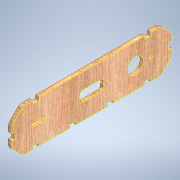
# Autodesk Inventor part: side
Saved by Autodesk Inventor 2020 (Build 240168000, 168)
## iProperties
Created: 2020-02-17
Part Number: side
Material: Wood (Birch)
Document SubType Name: Modeling
Designer: erwin
Density: 0.55 g/cm^3
Appearance: Birch - Natural Polished
Author: erwin
Autodesk Inventor part; units mm, degrees
ref_plane "YZ Plane" through (0, 0, 0) normal (1, 0, 0) x (0, 1, 0)
ref_plane "XZ Plane" through (0, 0, 0) normal (0, 1, 0) x (-1, 0, 0)
ref_plane "XY Plane" through (0, 0, 0) normal (0, 0, 1) x (1, 0, 0)
sketch "Sketch1" plane through (0, 0, 0) normal (1, 0, 0) x (0, 1, 0)
  line L0 (37.5736, 300) -> (-37.5736, 300)
  line L1 (-37.5736, 300) -> (-80, 257.5736)
  line L2 (-80, 257.5736) -> (-80, -257.5736)
  line L3 (-80, -257.5736) -> (-37.5736, -300)
  line L4 (-37.5736, -300) -> (37.5736, -300)
  line L5 (80, 257.5736) -> (80, -257.5736)
  line L6 (13.6652, 0) -> (-15.1656, 0) construction
  line L7 (0, 10.5835) -> (0, -18.7754) construction
  circle A0 centre (0, -220) radius 6
  line L8 (-0.0152, 220) -> (-0.0152, 180) construction
  line L9 (-6.0152, 220) -> (-6.0152, 180)
  line L10 (5.9848, 180) -> (5.9848, 220)
  arc A1 (5.9848, 220) -> (-6.0152, 220) centre (-0.0152, 220) ccw
  arc A2 (-6.0152, 180) -> (5.9848, 180) centre (-0.0152, 180) ccw
  line L11 (37.5736, 300) -> (80, 257.5736)
  line L12 (80, -257.5736) -> (37.5736, -300)
  circle A3 centre (-0.0152, -164) radius 30
  point P0 (0, 0)
  point P1 (80, 300)
  point P2 (80, -300)
  point P3 (-0.0152, 200)
  dimension "d0" = 160
  dimension "d1" = 45
  dimension "d2" = 12
  dimension "d3" = 40
  dimension "d4" = 12
  dimension "d5" = 400
  dimension "d6" = 80
  dimension "d7" = 80
  dimension "d8" = 80
  dimension "d9" = 80
  dimension "d10" = 60
  dimension "d15" = 60
  dimension "d16" = 60
  dimension "d17" = 45
  dimension "d18" = 56
  dimension "d19" = 60
  constraints: 28 end point, 4 centre point, 4 point on circle, 4 point on line, 4 tangent, 3 horizontal, 2 equal length, 2 parallel, 2 perpendicular, 2 vertical, 1 midpoint, 2 other
  measures "d0" distance between parallel lines of L5 L2
  measures "d1" angle of L4 L3
  measures "d2" diameter of A0
  measures "d3" distance of L8.start L8.end
  measures "d4" diameter of A2
  measures "d5" distance of A0.centre L8.end
  measures "d6" distance from line of L5 A0.centre
  measures "d7" distance from line of A0.centre L4
  measures "d8" distance from line of L2 A0.centre
  measures "d9" distance from line of L0 L8.start
  measures "d10" distance of L0.end L1.end
  measures "d15" distance of L0.start L5.start
  measures "d16" distance of L5.end L4.end
  measures "d17" angle of L5 L12
  measures "d18" distance of A0.centre A3.centre
  measures "d19" diameter of A3
extrude "Extrusion1" add sketch "Sketch1" along normal blind 12
fillet "Fillet1" radius 24 2 edges at (6, 80, 257.5736) (6, 37.5736, 300)
mirror "Mirror1" about plane through (0, 0, 0) normal (0, 1, 0) of "Fillet1"
mirror "Mirror2" about plane through (0, 0, 0) normal (0, 0, 1) of "Fillet1", "Mirror1"
sketch "Sketch6" plane through (0, 80, 247.6325) normal (0, 1, 0) x (1, 0, 0)
  line L0 (0, 67.6325) -> (0, 27.6325) projected
  line L1 (0, 50.07) -> (12, 50.07)
  line L2 (12, 50.07) -> (12, 26.07)
  line L3 (12, 26.07) -> (0, 26.07)
  line L4 (0, 26.07) -> (0, 50.07)
  point P0 (0, 247.6325)
  dimension "d23" = 12
  dimension "d24" = 24
  constraints: 8 end point, 2 parallel, 1 horizontal, 1 perpendicular, 1 point on line
  measures "d23" distance of L2.end L3.end
  measures "d24" distance of L1.end L2.end
extrude "Extrusion2" cut sketch "Sketch6" against normal blind 12
sketch "Sketch7" plane through (0, 27.6325, 300) normal (0, 0, 1) x (1, 0, 0)
  line L0 (-12, -15.6325) -> (12, -15.6325)
  line L1 (12, -15.6325) -> (12, -39.6325)
  line L2 (12, -39.6325) -> (-12, -39.6325)
  line L3 (-12, -39.6325) -> (-12, -15.6325)
  line L4 (-12, -15.6325) -> (12, -39.6325) construction
  line L5 (12, -15.6325) -> (-12, -39.6325) construction
  point P0 (0, -27.6325)
  dimension "d27" = 24
  dimension "d28" = 24
  constraints: 12 end point, 2 midpoint, 2 parallel, 1 horizontal, 1 perpendicular
  measures "d27" distance of L1.end L2.end
  measures "d28" distance of L0.end L1.end
extrude "Extrusion3" cut sketch "Sketch7" against normal blind 12
mirror "Mirror3" about plane through (0, 0, 0) normal (0, 1, 0) of "Extrusion2"
mirror "Mirror4" about plane through (0, 0, 0) normal (0, 0, 1) of "Extrusion2", "Mirror3", "Extrusion3"
sketch "Sketch8" plane through (0, -80, 197.5625) normal (0, -1, 0) x (1, 0, 0)
  line L0 (12, 0) -> (12, -395.125) projected
  line L1 (0, 0) -> (0, -395.125) projected
  line L2 (12, -115.7083) -> (0, -115.7083)
  line L3 (0, -115.7083) -> (0, -139.7083)
  line L4 (0, -139.7083) -> (12, -139.7083)
  line L5 (12, -139.7083) -> (12, -115.7083)
  line L6 (12, 0) -> (0, 0) projected
  line L7 (0, -395.125) -> (12, -395.125) projected
  point P0 (0, -197.5625)
  dimension "d31" = 24
  dimension "d32" = 115.7083
  dimension "d33" = 255.4167
  constraints: 8 end point, 2 parallel, 2 point on line, 1 horizontal, 1 perpendicular
  measures "d31" distance of L3.end L2.end
  measures "d32" distance between parallel lines of L6 L2
  measures "d33" distance between parallel lines of L7 L4
extrude "Extrusion4" cut sketch "Sketch8" against normal blind 12 contours L0 L4 L1 L2
mirror "Mirror5" about plane through (0, 0, 0) normal (0, 0, 1) of "Extrusion4"
sketch "Sketch9" plane through (12, 0, 0) normal (1, 0, 0) x (0, 0, -1)
  line L0 (-45, -10) -> (-45, 10)
  line L1 (-35, 20) -> (35, 20)
  line L2 (45, 10) -> (45, -10)
  line L3 (35, -20) -> (-35, -20)
  arc A0 (-45, -10) -> (-35, -20) centre (-35, -10) ccw
  arc A1 (45, 10) -> (35, 20) centre (35, 10) ccw
  arc A2 (35, -20) -> (45, -10) centre (35, -10) ccw
  arc A3 (-35, 20) -> (-45, 10) centre (-35, 10) ccw
  line L4 (0, 0) -> (0, 45.9772) construction
  line L5 (0, 0) -> (-28.8921, 0) construction
  point P0 (45, 20)
  point P1 (-45, 20)
  point P2 (45, -20)
  dimension "d36" = 40
  dimension "d37" = 90
  dimension "d38" = 10
  constraints: 12 end point, 8 point on circle, 8 tangent, 6 point on line, 4 centre point, 3 equal radius, 2 parallel, 1 horizontal, 1 perpendicular, 1 vertical, 2 other
  measures "d36" distance of point (45, 20) point (45, -20)
  measures "d37" distance of point (-45, 20) point (45, 20)
  measures "d38" radius of A0
extrude "Extrusion5" cut sketch "Sketch9" against normal through all
sketch "Sketch10" plane through (12, 0, 0) normal (1, 0, 0) x (0, 0, -1)
  arc A0 (-35, 20) -> (-45, 10) centre (-35, 10) ccw projected
  line L0 (-35, 20) -> (35, 20) projected
  arc A1 (45, 10) -> (35, 20) centre (35, 10) ccw projected
  line L1 (45, 10) -> (45, -10) projected
  arc A2 (35, -20) -> (45, -10) centre (35, -10) ccw projected
  line L2 (35, -20) -> (-35, -20) projected
  arc A3 (-45, -10) -> (-35, -20) centre (-35, -10) ccw projected
  line L3 (-45, -10) -> (-45, 10) projected
  line L4 (81.8542, -68) -> (81.8542, -80) projected
  line L5 (81.8542, -80) -> (197.5625, -80) projected
  line L6 (197.5625, -80) -> (197.5625, -68) projected
  line L7 (197.5625, -68) -> (221.5625, -68) projected
  line L8 (221.5625, -68) -> (221.5625, -80) projected
  line L9 (221.5625, -80) -> (247.6325, -80) projected
  arc A4 (247.6325, -80) -> (264.603, -72.9706) centre (247.6325, -56) ccw projected
  line L10 (264.603, -72.9706) -> (292.9706, -44.603) projected
  arc A5 (292.9706, -44.603) -> (300, -27.6325) centre (276, -27.6325) ccw projected
  line L11 (300, -27.6325) -> (300, -12) projected
  line L12 (300, -12) -> (288, -12) projected
  line L13 (288, -12) -> (288, 12) projected
  line L14 (288, 12) -> (300, 12) projected
  line L15 (300, 12) -> (300, 27.6325) projected
  arc A6 (300, 27.6325) -> (292.9706, 44.603) centre (276, 27.6325) ccw projected
  line L16 (292.9706, 44.603) -> (264.603, 72.9706) projected
  arc A7 (264.603, 72.9706) -> (247.6325, 80) centre (247.6325, 56) ccw projected
  line L17 (247.6325, 80) -> (221.5625, 80) projected
  line L18 (221.5625, 80) -> (221.5625, 68) projected
  line L19 (221.5625, 68) -> (197.5625, 68) projected
  line L20 (197.5625, 68) -> (197.5625, 80) projected
  line L21 (197.5625, 80) -> (-197.5625, 80) projected
  line L22 (-197.5625, 80) -> (-197.5625, 68) projected
  line L23 (-197.5625, 68) -> (-221.5625, 68) projected
  line L24 (-221.5625, 68) -> (-221.5625, 80) projected
  line L25 (-221.5625, 80) -> (-247.6325, 80) projected
  arc A8 (-247.6325, 80) -> (-264.603, 72.9706) centre (-247.6325, 56) ccw projected
  line L26 (-264.603, 72.9706) -> (-292.9706, 44.603) projected
  arc A9 (-292.9706, 44.603) -> (-300, 27.6325) centre (-276, 27.6325) ccw projected
  line L27 (-300, 27.6325) -> (-300, 12) projected
  line L28 (-300, 12) -> (-288, 12) projected
  line L29 (-288, 12) -> (-288, -12) projected
  line L30 (-288, -12) -> (-300, -12) projected
  line L31 (-300, -12) -> (-300, -27.6325) projected
  arc A10 (-300, -27.6325) -> (-292.9706, -44.603) centre (-276, -27.6325) ccw projected
  line L32 (-292.9706, -44.603) -> (-264.603, -72.9706) projected
  arc A11 (-264.603, -72.9706) -> (-247.6325, -80) centre (-247.6325, -56) ccw projected
  line L33 (-247.6325, -80) -> (-221.5625, -80) projected
  line L34 (-221.5625, -80) -> (-221.5625, -68) projected
  line L35 (-221.5625, -68) -> (-197.5625, -68) projected
  line L36 (-197.5625, -68) -> (-197.5625, -80) projected
  line L37 (-197.5625, -80) -> (-81.8542, -80) projected
  line L38 (-81.8542, -80) -> (-81.8542, -68) projected
  line L39 (-81.8542, -68) -> (-57.8542, -68) projected
  line L40 (-57.8542, -68) -> (-57.8542, -80) projected
  line L41 (-57.8542, -80) -> (57.8542, -80) projected
  line L42 (57.8542, -80) -> (57.8542, -68) projected
  line L43 (57.8542, -68) -> (81.8542, -68) projected
  circle A12 centre (220, 0) radius 6 projected
  circle A13 centre (164, -0.0152) radius 30 projected
  arc A14 (-180, -6.0152) -> (-180, 5.9848) centre (-180, -0.0152) ccw projected
  line L44 (-180, -6.0152) -> (-220, -6.0152) projected
  arc A15 (-220, 5.9848) -> (-220, -6.0152) centre (-220, -0.0152) ccw projected
  line L45 (-220, 5.9848) -> (-180, 5.9848) projected
  point P0 (0, 0)
equation "\"d7\" = d6"
equation "\"d8\" = d6"
equation "\"d9\" = d6"
equation "\"d15\" = d10"
equation "\"d16\" = d10"
equation "\"d17\" = d1"
equation "\"d32\" = -0.5 * d31 + 0.5 * d33"
body "Solid1"
